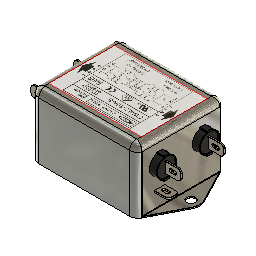
CW4EL2-10A-T EMI v2 (Autodesk Fusion 360 design; units mm, degrees)
Autodesk Fusion 360 part; units mm, degrees
note: some values were not read from the file. Chosen so that the rebuilt part matches the saved one: which bodies a step acts on.
sketch "Skizze1" plane through (0, 0, 0) normal (0, 0, 1) x (1, 0, 0)
  line L0 (-27, 26) -> (27, 26)
  arc A0 (31.439658, 23.299878) -> (27, 26) centre (27, 21) ccw
  line L1 (31.439658, 23.299878) -> (41.603453, 3.679805)
  arc A1 (41.603453, -3.679805) -> (41.603453, 3.679805) centre (34.5, 0) ccw
  line L2 (41.603453, -3.679805) -> (31.439658, -23.299878)
  arc A2 (27, -26) -> (31.439658, -23.299878) centre (27, -21) ccw
  line L3 (27, -26) -> (-27, -26)
  arc A3 (-31.439658, -23.299878) -> (-27, -26) centre (-27, -21) ccw
  line L4 (-31.439658, -23.299878) -> (-41.603453, -3.679805)
  arc A4 (-41.603453, 3.679805) -> (-41.603453, -3.679805) centre (-34.5, 0) ccw
  line L5 (-41.603453, 3.679805) -> (-31.439658, 23.299878)
  arc A5 (-27, 26) -> (-31.439658, 23.299878) centre (-27, 21) ccw
  line L6 (0, 0) -> (105.519236, 0) construction
  line L7 (0, 0) -> (0, 61.600377) construction
  line L8 (27, 21) -> (-27, 21) construction
  line L9 (-27, 21) -> (-27, -21) construction
  line L10 (-27, -21) -> (27, -21) construction
  line L11 (27, -21) -> (27, 21) construction
  line L12 (27, 21) -> (-27, -21) construction
  line L13 (-27, 21) -> (27, -21) construction
  circle A6 centre (37.5, 0) radius 2.5
  circle A7 centre (-37.5, 0) radius 2.5
  line L14 (-31.5, 23.183394) -> (-31.5, -23.183394)
  line L15 (31.5, 23.183394) -> (31.5, -23.183394)
  arc A8 (-30.511475, -23.304244) -> (-27, -25.2) centre (-27, -21) ccw
  line L16 (27, -25.2) -> (-27, -25.2)
  arc A9 (27, -25.2) -> (30.54375, -23.254293) centre (27, -21) ccw
  arc A10 (30.54375, 23.254293) -> (27, 25.2) centre (27, 21) ccw
  line L17 (-27, 25.2) -> (27, 25.2)
  arc A11 (-27, 25.2) -> (-30.54375, 23.254293) centre (-27, 21) ccw
  line L18 (-30.7, 22.717556) -> (-30.7, -22.67332)
  line L19 (30.7, 22.717556) -> (30.7, -22.717556)
  arc A12 (30.54375, -23.254293) -> (30.7, -22.717556) centre (29.7, -22.717556) ccw
  arc A13 (30.7, 22.717556) -> (30.54375, 23.254293) centre (29.7, 22.717556) ccw
  arc A14 (-30.54375, 23.254293) -> (-30.7, 22.717556) centre (-29.7, 22.717556) ccw
  arc A15 (-30.7, -22.67332) -> (-30.511475, -23.304244) centre (-29.55, -22.67332) ccw
  dimension "d7" = 5
  dimension "d8" = 8
  dimension "d9" = 52
  dimension "d10" = 5
  dimension "d13" = 5
  dimension "d14" = 37.5
  dimension "d15" = 69
  dimension "d16" = 34.5
  dimension "d17" = 37.5
  dimension "d18" = 31.5
  dimension "d19" = 27
  dimension "d65" = 1
  dimension "d66" = 1.15
  dimension "d67" = 0.8
  dimension "d68" = 0.8
  dimension "d69" = 0.8
  dimension "d70" = 0.8
  measures "d7" radius of A5
  measures "d8" radius of A4
  measures "d9" distance of L0 L3
  measures "d10" radius of A2
  measures "d13" diameter of A6
  measures "d65" radius of A12
  measures "d66" radius of A15
  measures "d67" distance of L3 L16
  measures "d68" distance of L0 L17
  measures "d69" distance of L14 L18
  measures "d70" distance of L15 L19
extrude "Extrusion1" add sketch "Skizze1" along normal blind 0.8 contours L0 A0 L1 L2 A2 L3 A3 L4 L5 A5 L14 L15 | L4 A4 L5 L14 | L1 A1 L2 L15 | A8 L16 A9 A10 L17 A11 L18 L19 A12 A13 A14 A15 picked at (-31.233333, -7.557773) picked at (-36.805542, 9.785403) picked at (36.805542, -9.785403) picked at (-9, -8.4) makes body 1
extrude "Extrusion2" add sketch "Skizze1" along normal blind 38 contours L0 A0 L1 L2 A2 L3 A3 L4 L5 A5 L14 L15 | A8 L16 A9 A10 L17 A11 L18 L19 A12 A13 A14 A15 picked at (-31.233333, -7.557773) picked at (-9, -8.4) bodies 1
fillet "Abrundung1" radius 4 12 edges at (-31.469829, -23.241636, 38) (-29.598135, -25.271966, 38) (0, -26, 38) (29.598135, -25.271966, 38) (31.469829, -23.241636, 38) (31.5, 0, 38) (31.469829, 23.241636, 38) (29.598135, 25.271966, 38) (0, 26, 38) (-29.598135, 25.271966, 38) (-31.469829, 23.241636, 38) (-31.5, 0, 38) on bodies 1
sketch "Skizze2" plane through (31.5, 0, 0) normal (1, 0, 0) x (0, 1, 0)
  line L0 (23.183394, 34) -> (-23.183394, 34)
  line L1 (-23.183394, 34) -> (-23.183394, 0.8)
  line L2 (-23.183394, 0.8) -> (23.183394, 0.8)
  line L3 (23.183394, 0.8) -> (23.183394, 34)
  line L4 (-12.25, 19.8) -> (-13.25, 19.8)
  line L5 (-13.25, 19.8) -> (-13.25, 26.2)
  line L6 (-13.25, 26.2) -> (-12.25, 26.2)
  line L7 (-12.25, 26.2) -> (-12.25, 19.8)
  line L8 (-12.25, 19.8) -> (-13.25, 26.2) construction
  line L9 (-13.25, 19.8) -> (-12.25, 26.2) construction
  line L10 (0, 0) -> (0, 41.520043) construction
  line L11 (-3.679805, 0) -> (-23.299878, 0) construction
  line L12 (12.25, 19.8) -> (13.25, 19.8)
  line L13 (12.25, 19.8) -> (13.25, 26.2) construction
  line L14 (13.25, 26.2) -> (12.25, 26.2)
  line L15 (13.25, 19.8) -> (12.25, 26.2) construction
  line L16 (12.25, 26.2) -> (12.25, 19.8)
  line L17 (13.25, 19.8) -> (13.25, 26.2)
  circle A0 centre (-12.75, 23) radius 5.4
  circle A1 centre (12.75, 23) radius 5.4
  line L18 (-9.55, 9.5) -> (-15.95, 9.5)
  line L19 (-15.95, 9.5) -> (-15.95, 10.5)
  line L20 (-15.95, 10.5) -> (-9.55, 10.5)
  line L21 (-9.55, 10.5) -> (-9.55, 9.5)
  line L22 (-9.55, 9.5) -> (-15.95, 10.5) construction
  line L23 (-15.95, 9.5) -> (-9.55, 10.5) construction
  line L24 (-11.15, 16.5) -> (-14.35, 16.5)
  line L25 (-14.35, 29.5) -> (-11.15, 29.5)
  line L26 (-11.15, 16.5) -> (-14.35, 29.5) construction
  line L27 (-14.35, 16.5) -> (-11.15, 29.5) construction
  line L28 (-14.35, 16.5) -> (-14.35, 17.217267)
  line L29 (-14.35, 28.782733) -> (-14.35, 29.5)
  line L30 (-11.15, 29.5) -> (-11.15, 28.782733)
  line L31 (-11.15, 17.217267) -> (-11.15, 16.5)
  arc A2 (-14.35, 28.782733) -> (-14.35, 17.217267) centre (-12.75, 23) ccw
  arc A3 (-11.15, 17.217267) -> (-11.15, 28.782733) centre (-12.75, 23) ccw
  line L32 (14.35, 16.5) -> (11.15, 16.5)
  line L33 (11.15, 29.5) -> (14.35, 29.5)
  line L34 (14.35, 16.5) -> (11.15, 29.5) construction
  line L35 (11.15, 16.5) -> (14.35, 29.5) construction
  line L36 (11.15, 16.5) -> (11.15, 17.217267)
  line L37 (11.15, 28.782733) -> (11.15, 29.5)
  line L38 (14.35, 29.5) -> (14.35, 28.782733)
  line L39 (14.35, 17.217267) -> (14.35, 16.5)
  arc A4 (11.15, 28.782733) -> (11.15, 17.217267) centre (12.75, 23) ccw
  arc A5 (14.35, 17.217267) -> (14.35, 28.782733) centre (12.75, 23) ccw
  dimension "d25" = 12.75
  dimension "d26" = 23
  dimension "d27" = 12
  dimension "d28" = 6.4
  dimension "d29" = 1
  dimension "d41" = 10.8
  dimension "d44" = 6.4
  dimension "d45" = 1
  dimension "d46" = 12.75
  dimension "d47" = 10
  dimension "d75" = 3.2
  dimension "d76" = 13
  dimension "d77" = 3.2
  dimension "d78" = 13
  measures "d25" distance of L10
  measures "d26" distance of L11
  measures "d27" diameter of A2
  measures "d41" diameter of A0
  measures "d46" distance of L10
  measures "d47" distance of L10.start
extrude "Extrusion3" add sketch "Skizze2" along normal blind 4.3 separate body contours L24 L25 L28 L29 L30 L31 A2 A3 | L32 L33 L36 L37 L38 L39 A4 A5 picked at (-12.884514, 16.8717) picked at (12.615486, 16.8717) makes body 2 at (34.366667, 18.123166, 22.462334) makes body 3 at (32.933333, -7.356713, 22.730832)
extrude "Extrusion4" add sketch "Skizze2" along normal blind 13 separate body contours L4 L5 L6 L7 | L12 L14 L16 L17 picked at (-12.916667, 24.066667) picked at (12.916667, 21.933333) makes body 4 at (35.833333, 12.25, 24.066667) makes body 5 at (35.833333, -13.25, 21.933333)
fillet "Abrundung2" radius 2 4 edges at (44.5, 12.75, 26.2) (44.5, 12.75, 19.8) (44.5, -12.75, 26.2) (44.5, -12.75, 19.8) on bodies 4 5
extrude "Extrusion10" add sketch "Skizze2" along normal blind 3.5 separate body contours A0 | A1 picked at (-14.883333, 23) picked at (10.616667, 23) makes body 6 at (32.666667, -7.376834, 22.462334) makes body 7 at (33.833333, 18.143287, 22.730832)
sketch "Skizze3" plane through (0, 13.25, 0) normal (0, 1, 0) x (-1, 0, 0)
  arc A0 (-44.5, 21.8) -> (-42.5, 19.8) centre (-42.5, 21.8) ccw
  line L0 (-42.5, 19.8) -> (-31.5, 19.8)
  line L1 (-31.5, 26.2) -> (-42.5, 26.2)
  arc A1 (-42.5, 26.2) -> (-44.5, 24.2) centre (-42.5, 24.2) ccw
  line L2 (-44.5, 24.2) -> (-44.5, 21.8)
  line L3 (-40.9, 22) -> (-38.7, 22)
  arc A2 (-38.7, 22) -> (-38.7, 24) centre (-38.7, 23) ccw
  line L4 (-38.7, 24) -> (-40.9, 24)
  arc A3 (-40.9, 24) -> (-40.9, 22) centre (-40.9, 23) ccw
  line L5 (-40.9, 23) -> (-38.7, 23) construction
  line L6 (-31.5, 19.8) -> (-31.5, 26.2)
  dimension "d36" = 2
  dimension "d37" = 3.2
  dimension "d38" = 2.2
  dimension "d55" = 3.6
  measures "d36" distance of L3 L4
  measures "d37" distance of L1 L5
  measures "d38" distance of origin
extrude "Extrusion5" cut sketch "Skizze3" against normal blind 26.5 contours L3 A2 L4 A3 picked at (-39.433333, 22.666667) bodies 4 5
extrude "Extrusion6" add sketch "Skizze2" along normal blind 3.8 separate body contours A0 | A1 picked at (-14.883333, 23) picked at (10.616667, 23) makes body 8 at (34.033333, -7.356713, 22.730832) makes body 9 at (34.033333, 18.143287, 22.730832)
fillet "Abrundung10" radius 0.1 8 edges at (33.65, 11.15, 29.5) (33.65, 14.35, 29.5) (33.65, 11.15, 16.5) (33.65, 14.35, 16.5) (33.65, -14.35, 29.5) (33.65, -11.15, 29.5) (33.65, -14.35, 16.5) (33.65, -11.15, 16.5) on bodies 2 3
fillet "Abrundung10" radius 0.1 8 edges at (33.65, 11.15, 17.217267) (33.65, 14.35, 17.217267) (33.65, 14.35, 28.782733) (33.65, 11.15, 28.782733) (33.65, -14.35, 28.782733) (33.65, -11.15, 28.782733) (33.65, -11.15, 17.217267) (33.65, -14.35, 17.217267) on bodies 2 3
fillet "Abrundung11" radius 0.1 34 edges at (35.8, 11.129959, 17.201727) (35.8, 11.15, 16.870836) (35.8, 11.179289, 16.529289) (35.8, 12.75, 16.5) (35.8, 14.320711, 16.529289) (35.8, 14.35, 16.870836) (35.8, 14.370041, 17.201727) (35.8, 18.75, 23) (35.8, 14.370041, 28.798273) (35.8, 14.35, 29.129164) (35.8, 14.320711, 29.470711) (35.8, 12.75, 29.5) (35.8, 11.179289, 29.470711) (35.8, 11.15, 29.129164) (35.8, 11.129959, 28.798273) (35.8, 6.75, 23) (35.8, 7.715432, 24.952723) (35.8, -14.370041, 17.201727) (35.8, -14.35, 16.870836) (35.8, -14.320711, 16.529289) (35.8, -12.75, 16.5) (35.8, -11.179289, 16.529289) (35.8, -11.15, 16.870836) (35.8, -11.129959, 17.201727) (35.8, -6.75, 23) (35.8, -11.129959, 28.798273) (35.8, -11.15, 29.129164) (35.8, -11.179289, 29.470711) (35.8, -12.75, 29.5) (35.8, -14.320711, 29.470711) (35.8, -14.35, 29.129164) (35.8, -14.370041, 28.798273) (35.8, -18.75, 23) (35.8, -17.784568, 24.952723) on bodies 2 3
mirror "Spiegeln1" about plane through (0, 0, 0) normal (1, 0, 0) of bodies 9 4 8 2 5 3 makes body 10 at (-38.833333, 12.583333, 19.8) makes body 11 at (-31.5, -14.883333, 23) makes body 12 at (-31.5, 10.616667, 23) makes body 13 at (-31.5, -12.916667, 24.066667) makes body 14 at (-34.3, 18.641038, 21.861725) makes body 15 at (-34.3, -6.858962, 21.861725)
extrude "Extrusion7" add sketch "Skizze2" along normal blind 8.5 separate body contours L18 L19 L20 L21 picked at (-11.683333, 9.833333) makes body 16
sketch "Skizze4" plane through (0, 0, 10.5) normal (0, 0, 1) x (-1, 0, 0)
  line L0 (-31.5, 9.55) -> (-31.5, 15.95)
  line L1 (-31.5, 15.95) -> (-40, 15.95)
  line L2 (-40, 15.95) -> (-40, 9.55)
  line L3 (-40, 9.55) -> (-31.5, 9.55)
  line L4 (-36.4, 11.75) -> (-34, 11.75)
  arc A0 (-34, 11.75) -> (-34, 13.75) centre (-34, 12.75) ccw
  line L5 (-34, 13.75) -> (-36.4, 13.75)
  arc A1 (-36.4, 13.75) -> (-36.4, 11.75) centre (-36.4, 12.75) ccw
  line L6 (-36.4, 12.75) -> (-34, 12.75) construction
  dimension "d50" = 2
  dimension "d51" = 3.6
  dimension "d52" = 2.4
  dimension "d56" = 3.2
  measures "d50" diameter of A0
  measures "d51" distance of L2
  measures "d56" distance of L1 L6
extrude "Extrusion8" cut sketch "Skizze4" against normal up to surface (1 mm away) contours L4 A0 L5 A1 picked at (-35.6, 12.416667) bodies 16
fillet "Abrundung3" radius 2 2 edges at (40, -15.95, 10) (40, -9.55, 10) on bodies 16
fillet "Abrundung4" radius 0.1 90 edges at (39.8, 12.25, 22) (37.7, 12.25, 23) (39.8, 12.25, 24) (41.9, 12.25, 23) (37, 12.25, 19.8) (43.914214, 12.25, 20.385786) (44.5, 12.25, 23) (43.914214, 12.25, 25.614214) (37, 12.25, 26.2) (39.8, 13.25, 22) (41.9, 13.25, 23) (39.8, 13.25, 24) (37.7, 13.25, 23) (37, 13.25, 19.8) (43.914214, 13.25, 20.385786) (44.5, 13.25, 23) (43.914214, 13.25, 25.614214) (37, 13.25, 26.2) (37, -13.25, 26.2) (43.914214, -13.25, 25.614214) (44.5, -13.25, 23) (43.914214, -13.25, 20.385786) (37, -13.25, 19.8) (37, -12.25, 26.2) (43.914214, -12.25, 25.614214) (44.5, -12.25, 23) (43.914214, -12.25, 20.385786) (37, -12.25, 19.8) (39.8, -13.25, 24) (41.9, -13.25, 23) (39.8, -13.25, 22) (37.7, -13.25, 23) (39.8, -12.25, 24) (37.7, -12.25, 23) (39.8, -12.25, 22) (41.9, -12.25, 23) (-39.8, 12.25, 22) (-37.7, 12.25, 23) (-39.8, 12.25, 24) (-41.9, 12.25, 23) (-37, 12.25, 26.2) (-43.914214, 12.25, 25.614214) (-44.5, 12.25, 23) (-43.914214, 12.25, 20.385786) (-37, 12.25, 19.8) (-37, 13.25, 19.8) (-43.914214, 13.25, 20.385786) (-44.5, 13.25, 23) (-43.914214, 13.25, 25.614214) (-37, 13.25, 26.2) (-39.8, 13.25, 22) (-41.9, 13.25, 23) (-39.8, 13.25, 24) (-37.7, 13.25, 23) (-39.8, -12.25, 22) (-41.9, -12.25, 23) (-39.8, -12.25, 24) (-37.7, -12.25, 23) (-37, -12.25, 26.2) (-43.914214, -12.25, 25.614214) (-44.5, -12.25, 23) (-43.914214, -12.25, 20.385786) (-37, -12.25, 19.8) (-37, -13.25, 26.2) (-43.914214, -13.25, 25.614214) (-44.5, -13.25, 23) (-43.914214, -13.25, 20.385786) (-37, -13.25, 19.8) (-39.8, -13.25, 22) (-37.7, -13.25, 23) (-39.8, -13.25, 24) (-41.9, -13.25, 23) (34.75, -15.95, 10.5) (39.414214, -15.364214, 10.5) (40, -12.75, 10.5) (39.414214, -10.135786, 10.5) (34.75, -9.55, 10.5) (34.75, -15.95, 9.5) (39.414214, -15.364214, 9.5) (40, -12.75, 9.5) (39.414214, -10.135786, 9.5) (34.75, -9.55, 9.5) (35.2, -13.75, 10.5) (33, -12.75, 10.5) (35.2, -11.75, 10.5) (37.4, -12.75, 10.5) (35.2, -13.75, 9.5) (37.4, -12.75, 9.5) (35.2, -11.75, 9.5) (33, -12.75, 9.5) on bodies 4 5 10 13 16
fillet "Abrundung5" radius 0.25 2 edges at (31.5, 0, 0.8) (-31.5, 0, 0.8) on bodies 1
fillet "Abrundung6" radius 0.1 16 edges at (29.598135, 25.271966, 0) (36.521555, 13.489841, 0) (42.5, 0, 0) (36.521555, -13.489841, 0) (29.598135, -25.271966, 0) (0, -26, 0) (-29.598135, -25.271966, 0) (-36.521555, -13.489841, 0) (-42.5, 0, 0) (-36.521555, 13.489841, 0) (-29.598135, 25.271966, 0) (0, 26, 0) (-39.830818, 0.904039, 0) (-39.830818, 0.904039, 0.8) (35.169182, 0.904039, 0.8) (35.169182, 0.904039, 0) on bodies 1
fillet "Abrundung7" radius 0.1 22 edges at (29.41841, -22.633583, 37.509923) (31.363045, -23.150026, 35.037728) (31.5, -23.183394, 17.525) (31.573223, -23.042045, 0.873223) (36.676726, -13.190301, 0.8) (42.5, 0, 0.8) (36.676726, 13.190301, 0.8) (31.573223, 23.042045, 0.873223) (31.5, 23.183394, 17.525) (31.363045, 23.150026, 35.037728) (29.41841, 22.633583, 37.509923) (-29.41841, 22.633583, 37.509923) (-31.363045, 23.150026, 35.037728) (-31.5, 23.183394, 17.525) (-31.573223, 23.042045, 0.873223) (-36.676726, 13.190301, 0.8) (-42.5, 0, 0.8) (-36.676726, -13.190301, 0.8) (-31.573223, -23.042045, 0.873223) (-31.5, -23.183394, 17.525) (-31.363045, -23.150026, 35.037728) (-29.41841, -22.633583, 37.509923) on bodies 1
extrude "Extrusion9" cut sketch "Skizze1" along normal blind 0.3 contours A8 L16 A9 A10 L17 A11 L18 L19 A12 A13 A14 A15 picked at (-9, -8.4) bodies 1
fillet "Abrundung8" radius 0.2 12 edges at (30.660143, -22.997065, 0.3) (30.7, 0, 0.3) (30.660143, 22.997065, 0.3) (29.021382, 24.681578, 0.3) (0, 25.2, 0.3) (-29.021382, 24.681578, 0.3) (-30.660143, 22.997065, 0.3) (-30.7, 0.022118, 0.3) (-30.651861, -23.002564, 0.3) (-28.995266, -24.695797, 0.3) (0, -25.2, 0.3) (29.021382, -24.681578, 0.3) on bodies 1
fillet "Abrundung9" radius 0.1 12 edges at (30.660143, -22.997065, 0) (30.7, 0, 0) (30.660143, 22.997065, 0) (29.021382, 24.681578, 0) (0, 25.2, 0) (-29.021382, 24.681578, 0) (-30.660143, 22.997065, 0) (-30.7, 0.022118, 0) (-30.651861, -23.002564, 0) (-28.995266, -24.695797, 0) (0, -25.2, 0) (29.021382, -24.681578, 0) on bodies 1
equation "d14 = ( 75 / 2 ) * 1 mm"
equation "d16 = d15 / 2"
equation "d17 = d14"
equation "d18 = ( 63 / 2 ) * 1 mm"
equation "d25 = ( 25.5 / 2 ) * 1 mm"
equation "d44 = d28"
equation "d45 = d29"
equation "d46 = d25"
equation "d79 = 4.3 mm - 0.8 mm"
